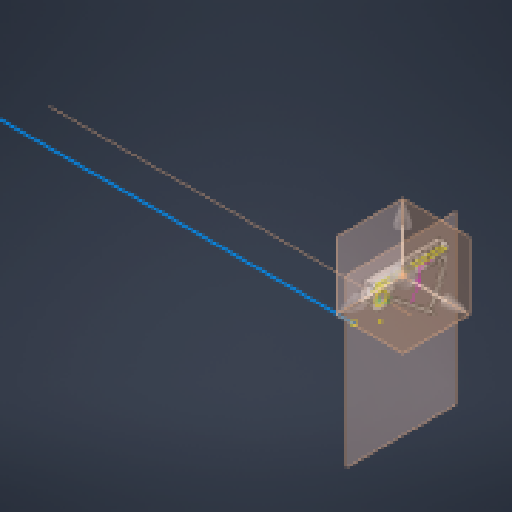
# Autodesk Inventor part: sensor arm v3
Saved by Autodesk Inventor 2025 (Build 290162000, 162)
## iProperties
Created: 2022-06-07
Part Number: sensor arm v3
Material: Generic
Document SubType Name: Modeling
Designer: micha
Density: 1 g/cm^3
Appearance: Default
Mass: 4.64954 g
Surface Area: 36.1007 cm^2
Volume: 4.64954 cm^3
Author: micha
Autodesk Inventor part; units mm, degrees
ref_plane "YZ Plane" through (0, 0, 0) normal (1, 0, 0) x (0, 1, 0)
ref_plane "XZ Plane" through (0, 0, 0) normal (0, 1, 0) x (-1, 0, 0)
ref_plane "XY Plane" through (0, 0, 0) normal (0, 0, 1) x (1, 0, 0)
ref_plane "Work Plane1" through (2.8939, -10.5569, -51.7376) normal (1, 0, 0) x (0, 0, -1)
sketch "Sketch1" plane through (2.8939, -10.5569, -51.7376) normal (1, 0, 0) x (0, 0, -1)
  line L0 (1, 38.5569) -> (1, -0.3026)
  spline S0 degree 2 poles (-6.3132, 4.7596) (-27.3933, 12.7232) (-66.3273, 26.8684) knots 1.083719 1.083719 1.083719 7.262987 7.262987 7.262987 weights 1.016219 1.054601 1.003399
  spline S1 degree 2 poles (-66, 24.0035) (-21.1228, 7.8362) (0, 0) knots 0 0 0 7.022956 7.022956 7.022956 weights 1 1.068995 1
  circle A0 centre (-63, 31.2793) radius 2.05
  circle A1 centre (-39, 31.2793) radius 2.05
  circle A2 centre (-27, 19.2793) radius 2.05
  circle A3 centre (-21, 25.2793) radius 2.05
  circle A4 centre (-15, 25.2793) radius 2.05
  circle A5 centre (-15, 19.2793) radius 2.05
  circle A6 centre (-21, 31.2793) radius 2.05
  circle A7 centre (-33, 19.2793) radius 2.05
  circle A8 centre (-45, 25.2793) radius 2.05
  circle A9 centre (-51, 31.2793) radius 2.05
  circle A10 centre (-51, 25.2793) radius 2.05
  circle A11 centre (-33, 25.2793) radius 2.05
  circle A12 centre (-27, 25.2793) radius 2.05
  circle A13 centre (-21, 19.2793) radius 2.05
  circle A14 centre (-15, 31.2793) radius 2.05
  circle A15 centre (-39, 25.2793) radius 2.05
  circle A16 centre (-15, 13.2793) radius 2.05
  circle A17 centre (-27, 31.2793) radius 2.05
  circle A18 centre (-33, 31.2793) radius 2.05
  circle A19 centre (-45, 31.2793) radius 2.05
  circle A20 centre (-57, 31.2793) radius 2.05
  line L1 (-6.3132, 20.0885) -> (-9, 20.0885)
  line L2 (-9, 20.0885) -> (-9, 22.0793)
  line L3 (-9, 22.0793) -> (-6.3132, 22.0793)
  line L4 (-6.3132, 22.0793) -> (-6.3132, 26.0885)
  line L5 (-6.3132, 26.0885) -> (-9, 26.0885)
  line L6 (-9, 26.0885) -> (-9, 28.0793)
  line L7 (-9, 28.0793) -> (-6.3132, 28.0793)
  line L8 (-6.3132, 28.0793) -> (-6.3132, 32.0885)
  line L9 (-6.3132, 32.0885) -> (-9, 32.0885)
  line L10 (-9, 32.0885) -> (-9, 34.0793)
  line L11 (-9, 34.0793) -> (-6.3132, 34.0793)
  line L12 (-6.3132, 34.0793) -> (-6.3132, 38.0885)
  line L13 (-6.3132, 38.0885) -> (-9, 38.0885)
  line L14 (-9, 38.0885) -> (-9, 38.5569)
  line L15 (-9, 38.5569) -> (-69, 38.5569)
  line L16 (-69, 38.5569) -> (-69, 26.0323)
  spline S2 degree 3 poles (-68.9282, 25.4918) (-68.9763, 25.6696) (-69, 25.8616) (-69, 26.0323) knots 0 0 0 0 1 1 1 1
  line L17 (-6.3132, 4.7596) -> (-6.3132, 8.0885)
  line L18 (-6.3132, 8.0885) -> (-9, 8.0885)
  line L19 (-9, 8.0885) -> (-9, 10.0793)
  line L20 (-9, 10.0793) -> (-6.3132, 10.0793)
  line L21 (-6.3132, 10.0793) -> (-6.3132, 14.0885)
  line L22 (-6.3132, 14.0885) -> (-9, 14.0885)
  line L23 (-9, 14.0885) -> (-9, 16.0793)
  line L24 (-9, 16.0793) -> (-6.3132, 16.0793)
  line L25 (-6.3132, 16.0793) -> (-6.3132, 20.0885)
  circle A21 centre (-51, 25.2793) radius 51
  line L26 (-69, 43.5569) -> (1, 43.5569)
  line L27 (0, 25.2793) -> (0, 43.5569)
  circle A22 centre (-63, 31.2793) radius 2.05
  circle A23 centre (-39, 31.2793) radius 2.05
  circle A24 centre (-27, 19.2793) radius 2.05
  circle A25 centre (-21, 25.2793) radius 2.05
  circle A26 centre (-15, 25.2793) radius 2.05
  circle A27 centre (-15, 19.2793) radius 2.05
  circle A28 centre (-21, 31.2793) radius 2.05
  circle A29 centre (-33, 19.2793) radius 2.05
  circle A30 centre (-45, 25.2793) radius 2.05
  circle A31 centre (-51, 31.2793) radius 2.05
  circle A32 centre (-51, 25.2793) radius 2.05
  circle A33 centre (-33, 25.2793) radius 2.05
  circle A34 centre (-27, 25.2793) radius 2.05
  circle A35 centre (-21, 19.2793) radius 2.05
  circle A36 centre (-15, 31.2793) radius 2.05
  circle A37 centre (-39, 25.2793) radius 2.05
  circle A38 centre (-15, 13.2793) radius 2.05
  circle A39 centre (-27, 31.2793) radius 2.05
  circle A40 centre (-33, 31.2793) radius 2.05
  circle A41 centre (-45, 31.2793) radius 2.05
  circle A42 centre (-57, 31.2793) radius 2.05
  line L28 (0, 3.2928) -> (0, 0)
  line L29 (-66, 43.5569) -> (-66, 24.0035)
  line L30 (-7.9338, 43.5569) -> (-66, 43.5569)
  line L31 (1, 3.5569) -> (1, 2.9251)
  spline S3 degree 2 poles (0, 3.2928) (0.5038, 3.1076) (1, 2.9251) knots 0 0 0 1 1 1 weights 1.002419 1.001235 1
  line L32 (-5.5888, 2.0667) -> (-8.7079, -13.6264)
  line L33 (-51, 25.2793) -> (1.0658, -16.3025)
  line L34 (-49.7207, 26.8812) -> (1, -13.6264)
  circle A43 centre (-51, 25.2793) radius 57.952
  circle A44 centre (-51, 25.2793) radius 49.5
  circle A45 centre (-51, 25.2793) radius 5
  line L35 (-51, 30.2793) -> (1, 30.2793)
  line L36 (-51, 28.5561) -> (1, 28.5561)
  line L37 (-6, 27.6203) -> (1, 27.6203)
  line L38 (1, 30.1203) -> (1, 27.6203)
  line L39 (1, 30.1203) -> (-7, 30.1203)
  line L40 (-7, 24.1203) -> (-7, 30.1203)
  line L41 (1, 24.1203) -> (-7, 24.1203)
  line L42 (1, 26.6203) -> (1, 24.1203)
  line L43 (1, 26.6203) -> (-6, 26.6203)
  line L44 (-6, 26.6203) -> (-6, 27.6203)
  line L45 (1, 43.5569) -> (1, -27.3438)
  circle A46 centre (-51, 25.2793) radius 3
  line L46 (-7.9338, 3.5569) -> (1, 3.5569)
  spline S4 degree 3 poles (-68.9282, 25.4918) (-68.9051, 25.5773) (-68.8768, 25.6596) (-68.7507, 25.9672) (-68.5854, 26.218) (-68.2351, 26.5719) (-67.989, 26.7385) (-67.5342, 26.9287) (-67.2454, 26.9869) (-67, 26.9869) (-66.8321, 26.9869) (-66.6438, 26.9597) (-66.4687, 26.9138) knots 0 0 0 0 0.082605 0.082605 0.334613 0.334613 0.583858 0.583858 0.830936 0.830936 0.830936 1 1 1 1
  line L47 (-67.3682, 24.0029) -> (-66.4687, 26.9138)
  spline S5 degree 2 poles (-67.3682, 24.0029) (-63.8358, 22.7167) (-60.4985, 21.4988) knots 0.11627 0.11627 0.11627 0.626298 0.626298 0.626298 weights 1.002483 1.007844 1.012449
  line L48 (-60.1926, 22.4888) -> (-60.4985, 21.4988)
  line L49 (-60.273, 22.4962) -> (-60.1926, 22.4888)
  line L50 (-61.0288, 24.942) -> (-60.273, 22.4962)
  spline S6 degree 2 poles (-57.0533, 23.4947) (-59.0095, 24.2073) (-61.0288, 24.942) knots 0 0 0 1 1 1 weights 1.014246 1.01214 1.009793
  line L51 (-57.4032, 22.3623) -> (-57.0533, 23.4947)
  line L52 (-56.7087, 20.1148) -> (-57.4032, 22.3623)
  spline S7 degree 2 poles (-56.7087, 20.1148) (-54.1005, 19.1616) (-51.6095, 18.2493) knots 0 0 0 1 1 1 weights 1.017547 1.020956 1.023858
  line L53 (-50.7041, 21.1795) -> (-51.6095, 18.2493)
  spline S8 degree 2 poles (-47.3081, 19.939) (-48.981, 20.5505) (-50.7041, 21.1795) knots 0 0 0 1 1 1 weights 1.023609 1.022223 1.020626
  line L54 (-46.1695, 16.2542) -> (-47.3081, 19.939)
  spline S9 degree 2 poles (-46.1695, 16.2542) (-44.6707, 15.7038) (-43.2153, 15.1685) knots 0 0 0 1 1 1 weights 1.029758 1.031251 1.032536
  line L55 (-42.3067, 18.1089) -> (-43.2153, 15.1685)
  spline S10 degree 2 poles (-37.3514, 16.2915) (-39.7706, 17.1799) (-42.3067, 18.1089) knots 0 0 0 1 1 1 weights 1.030206 1.029053 1.02736
  line L56 (-36.2059, 12.5846) -> (-37.3514, 16.2915)
  spline S11 degree 2 poles (-36.2059, 12.5846) (-35.7451, 12.4143) (-35.2889, 12.2456) knots 0 0 0 1 1 1 weights 1.037681 1.037944 1.038183
  line L57 (-34.3765, 15.1982) -> (-35.2889, 12.2456)
  spline S12 degree 2 poles (-31.8369, 14.2634) (-33.0902, 14.7251) (-34.3765, 15.1982) knots 0 0 0 1 1 1 weights 1.032167 1.031883 1.031435
  line L58 (-32.7507, 11.3063) -> (-31.8369, 14.2634)
  spline S13 degree 2 poles (-32.7507, 11.3063) (-31.3433, 10.7849) (-29.9802, 10.2787) knots 0 0 0 1 1 1 weights 1.039335 1.039874 1.040168
  line L59 (-31.1312, 14.0034) -> (-29.9802, 10.2787)
  spline S14 degree 2 poles (-27.9388, 12.8256) (-29.5079, 13.4052) (-31.1312, 14.0034) knots 0 0 0 1 1 1 weights 1.03266 1.032626 1.032315
  line L60 (-27.3534, 10.9314) -> (-27.9388, 12.8256)
  line L61 (-26.888, 12.4374) -> (-27.3534, 10.9314)
  spline S15 degree 2 poles (-24.3498, 11.4984) (-25.601, 11.9617) (-26.888, 12.4374) knots 0 0 0 1 1 1 weights 1.03236 1.032601 1.032651
  line L62 (-25.2685, 8.5253) -> (-24.3498, 11.4984)
  spline S16 degree 2 poles (-25.2685, 8.5253) (-23.1143, 7.7218) (-21.0732, 6.9569) knots 0 0 0 1 1 1 weights 1.040431 1.040189 1.039256
  line L63 (-22.2343, 10.7144) -> (-21.0732, 6.9569)
  spline S17 degree 2 poles (-17.2807, 8.8727) (-19.6843, 9.7684) (-22.2343, 10.7144) knots 2.532276 2.532276 2.532276 3.127294 3.127294 3.127294 weights 1.029291 1.030965 1.031808
  line L64 (-18.0732, 6.3082) -> (-17.2807, 8.8727)
  line L65 (-17.9038, 5.7667) -> (-18.0732, 6.3082)
  spline S18 degree 2 poles (-17.9038, 5.7667) (-15.9349, 5.0258) (-14.071, 4.3204) knots 0 0 0 1 1 1 weights 1.037347 1.035864 1.033687
  line L66 (-13.4423, 6.3549) -> (-14.071, 4.3204)
  line L67 (-13.8213, 7.5812) -> (-13.4423, 6.3549)
  spline S19 degree 2 poles (-10.6072, 6.3767) (-12.1801, 6.9674) (-13.8213, 7.5812) knots 0 0 0 1 1 1 weights 1.022735 1.024771 1.02639
  line L68 (-10.6139, 6.3549) -> (-10.6072, 6.3767)
  line L69 (-9.4416, 2.5612) -> (-10.6139, 6.3549)
  spline S20 degree 2 poles (-9.4416, 2.5612) (-8.5985, 2.2395) (-7.7778, 1.9252) knots 0 0 0 1 1 1 weights 1.026979 1.025506 1.023872
  line L70 (-6.8404, 4.9587) -> (-7.7778, 1.9252)
  spline S21 degree 2 poles (-6.3132, 4.7596) (-6.5758, 4.8589) (-6.8404, 4.9587) knots 0 0 0 1 1 1 weights 1.016219 1.01668 1.017128
  spline S22 degree 2 poles (-47.8503, 17.4555) (-47.0907, 17.181) (-46.3417, 16.9102) knots 0 0 0 1 1 1 weights 1.022634 1.023401 1.024117
  spline S23 degree 2 poles (-0.7385, 0.2738) (-0.3669, 0.1361) (0, 0) knots 0 0 0 1 1 1 weights 1.002208 1.001122 1
  spline S24 degree 2 poles (-0.7385, 0.2738) (-1.5648, 0.5801) (-2.4148, 0.8945) knots 0 0 0 1 1 1 weights 1.005252 1.007625 1.009817
  spline S25 degree 2 poles (-4.9534, 1.8323) (-3.6579, 1.3544) (-2.4148, 0.8945) knots 0 0 0 1 1 1 weights 1.01307 1.010167 1.006872
  spline S26 degree 2 poles (-4.9534, 1.8323) (-5.0001, 1.8495) (-5.0468, 1.8668) knots 0 0 0 1 1 1 weights 1.015865 1.015967 1.016069
  spline S27 degree 2 poles (-8.2385, 3.0424) (-6.6033, 2.4409) (-5.0468, 1.8668) knots 0 0 0 1 1 1 weights 1.019681 1.016766 1.013279
  spline S28 degree 2 poles (-8.2385, 3.0424) (-8.4827, 3.1322) (-8.7287, 3.2226) knots 0 0 0 1 1 1 weights 1.022285 1.022707 1.023117
  spline S29 degree 2 poles (-11.2688, 4.1555) (-9.9751, 3.6808) (-8.7287, 3.2226) knots 0 0 0 1 1 1 weights 1.024514 1.022693 1.020541
  spline S30 degree 2 poles (-11.2688, 4.1555) (-12.1147, 4.4658) (-12.9815, 4.7835) knots 0 0 0 1 1 1 weights 1.026945 1.02809 1.029093
  spline S31 degree 2 poles (-17.9571, 6.6037) (-15.3856, 5.6644) (-12.9815, 4.7835) knots 4.545675 4.545675 4.545675 5.174639 5.174639 5.174639 weights 1.031505 1.029685 1.026759
  spline S32 degree 2 poles (-17.9571, 6.6037) (-19.6666, 7.2282) (-21.4541, 7.8799) knots 0 0 0 1 1 1 weights 1.033564 1.034685 1.035312
  spline S33 degree 2 poles (-25.0396, 9.186) (-23.2077, 8.5192) (-21.4541, 7.8799) knots 0 0 0 1 1 1 weights 1.034382 1.034148 1.03344
  spline S34 degree 2 poles (-25.0396, 9.186) (-27.4467, 10.0621) (-29.9959, 10.9881) knots 3.443887 3.443887 3.443887 3.981642 3.981642 3.981642 weights 1.036069 1.036254 1.035617
  spline S35 degree 2 poles (-31.3054, 11.4637) (-30.6459, 11.2242) (-29.9959, 10.9881) knots 0 0 0 1 1 1 weights 1.033862 1.034046 1.034176
  spline S36 degree 2 poles (-31.3054, 11.4637) (-31.5323, 11.546) (-31.7603, 11.6288) knots 0 0 0 1 1 1 weights 1.035239 1.035165 1.035085
  spline S37 degree 2 poles (-33.4388, 12.2379) (-32.5919, 11.9307) (-31.7603, 11.6288) knots 0 0 0 1 1 1 weights 1.033138 1.033475 1.033729
  spline S38 degree 2 poles (-33.4388, 12.2379) (-35.6339, 13.0343) (-37.9355, 13.8682) knots 0 0 0 1 1 1 weights 1.034414 1.033438 1.0319
  spline S39 degree 2 poles (-39.3424, 14.3777) (-38.6339, 14.1212) (-37.9355, 13.8682) knots 0 0 0 1 1 1 weights 1.029908 1.030394 1.030829
  spline S40 degree 2 poles (-39.3424, 14.3777) (-40.1336, 14.6643) (-40.9376, 14.9553) knots 0 0 0 1 1 1 weights 1.030917 1.03034 1.029698
  spline S41 degree 2 poles (-42.8319, 15.6409) (-41.8759, 15.295) (-40.9376, 14.9553) knots 0 0 0 1 1 1 weights 1.027259 1.028053 1.02876
  spline S42 degree 2 poles (-42.8319, 15.6409) (-44.5572, 16.2651) (-46.3417, 16.9102) knots 0 0 0 1 1 1 weights 1.028117 1.026614 1.02483
  spline S43 degree 2 poles (-47.8503, 17.4555) (-49.2326, 17.9551) (-50.651, 18.4673) knots 0 0 0 1 1 1 weights 1.023286 1.021839 1.02023
  spline S44 degree 2 poles (-52.7716, 19.2331) (-51.7012, 18.8466) (-50.651, 18.4673) knots 0 0 0 1 1 1 weights 1.017303 1.01854 1.019688
  spline S45 degree 2 poles (-52.7716, 19.2331) (-53.9932, 19.6741) (-55.2416, 20.1246) knots 0 0 0 1 1 1 weights 1.017764 1.01631 1.01474
  spline S46 degree 2 poles (-56.8566, 20.7073) (-56.0435, 20.414) (-55.2416, 20.1246) knots 0 0 0 1 1 1 weights 1.012371 1.013395 1.014371
  spline S47 degree 2 poles (-56.8566, 20.7073) (-58.8593, 21.4298) (-60.9319, 22.177) knots 0 0 0 1 1 1 weights 1.012682 1.010099 1.00723
  spline S48 degree 2 poles (-63.2903, 23.0271) (-62.0997, 22.598) (-60.9319, 22.177) knots 0 0 0 1 1 1 weights 1.003834 1.005493 1.007062
  spline S49 degree 2 poles (-63.2903, 23.0271) (-63.9732, 23.2732) (-64.6637, 23.522) knots 0 0 0 1 1 1 weights 1.003923 1.002951 1.00195
  spline S50 degree 2 poles (-66, 24.0035) (-65.3283, 23.7615) (-64.6637, 23.522) knots 0 0 0 1 1 1 weights 1 1.000967 1.001907
  line L71 (-7.9338, 43.5569) -> (-7.9338, 3.5569)
  point P0 (-51.7376, 10.5569)
  point P1 (-4.4661, -9.261)
  point P2 (-5.717, -10.8854)
  point P3 (-11.0752, -3.9826)
  point P4 (-46.1572, 24.0352)
  point P5 (-47.2234, 28.5561)
  point P6 (-1.6086, 28.5561)
  point P7 (-0.2303, 30.1203)
  point P8 (-6.3132, 30.1203)
  point P9 (-6.3132, 30.2793)
  point P10 (-49.2104, 30.2793)
  point P11 (-49.3883, 30.0124)
  point P12 (-47.0931, 22.1591)
  point P13 (-11.1492, -6.5471)
  point P14 (-0.2457, 30.2793)
extrude "Thickness" add sketch "Sketch1" along normal mid plane 3 contours A21 L39 A44 L35 | A21 L36 A44 L39 | A44 L39 L8 L35 | L33 A44 L34 A21 | A21 L37 A44 L36 | A44 L36 L8 L39 | L8 L39 L40 L36 L71 L35 | L34 A44 S1 A21 | L33 L57 S1 L58 S13 L59 L34 A44 | A21 L43 A44 L37 | L8 L36 L40 L39 | L71 L36 A45 A9 L35 A19 A1 A18 A17 A6 A14 | S1 A44 L46 A21 | L33 S1 L57 | L41 A44 L43 A21 | A21 L46 A44 L41 | A14 L35 | S1 L59 L34 | L33 L56 S0 L34 L57 S1 | L57 L34 L58 S1 | A45 A8 L34 A46 L33 S0 A9 | L59 S1 L58 L34 | L33 S0 L56 | A6 L35 | A45 L34 A8 | A9 A45 | L59 S13 L58 S1 | L33 A45 A8 L34 S0 | L34 A45 A8 | A8 A45 L33 A46 L34 | A8 A45 L34 | A17 L35 | A46 L33 A10 L34 | L34 A10 L33 A46 | S0 L53 A45 | L35 A19 | A45 L53 S0 | A18 L35 | L35 A1 picked at (-15.4743, 29.9145) picked at (-21.4743, 29.9145) picked at (-46.3486, 25.5853) picked at (-46.6382, 24.3353) picked at (-45.6216, 23.5252) picked at (-27.4743, 29.9145) picked at (-44.8638, 29.6994) picked at (-32.9196, 29.6737) picked at (-38.8638, 29.6994)
sketch "Sketch2" plane through (1.3939, 19.7224, -2.5271) normal (0, 1, 0) x (1, 0, 0)
  line L0 (0, 0) -> (0, 48.9648) projected
  line L1 (0, 0) -> (3, 0) projected
  line L2 (3, 48.9648) -> (3, 0) projected
  line L3 (0, 48.9648) -> (3, 48.9648) projected
  line L4 (0, 2.1174) -> (0, -0.1779) projected
  line L5 (0, 2.1174) -> (3, 2.1174) projected
  line L6 (3, -0.1779) -> (3, 2.1174) projected
  line L7 (0, -0.1779) -> (3, -0.1779) projected
  line L8 (3, -6.7896) -> (3, 2.1174) projected
  line L9 (0, 49.2104) -> (0, 38.0612) projected
  line L10 (3, -6.7896) -> (0, -6.7896)
  line L11 (0, -6.7896) -> (0, 49.2104)
  line L12 (0, 49.2104) -> (3, 49.2104)
  line L13 (3, 49.2104) -> (3, -6.7896)
  point P0 (-1.3939, -2.5271)
  constraints: 8 end point, 2 parallel, 1 horizontal, 1 perpendicular
sketch "Sketch3" plane through (4.3939, -10.5569, -51.7376) normal (1, 0, 0) x (0, 0, -1)
  arc A0 (-11.1492, -6.5471) -> (-0.2457, 30.2793) centre (-51, 25.2793) ccw projected
  line L0 (-0.2457, 30.2793) -> (-47.7223, 30.2793)
  line L1 (-47.7223, 30.2793) -> (-47.7223, 24.2793)
  line L2 (-47.7223, 24.2793) -> (-0.2457, 24.2793)
  line L3 (-0.2457, 24.2793) -> (-0.2457, 30.2793)
  point P0 (-51.7376, 10.5569)
  dimension "d10" = 6
  constraints: 8 end point, 2 parallel, 1 horizontal, 1 perpendicular
  measures "d10" distance between parallel lines of L2 L0
extrude "sensor weight" [suppressed]
sketch "Sketch4" plane through (1.3939, 19.7224, -2.5271) normal (0, 1, 0) x (1, 0, 0)
  line L0 (0, 0) -> (3, 0) projected
  line L1 (3, 48.9648) -> (3, 0) projected
  line L2 (0, 48.9648) -> (3, 48.9648) projected
  line L3 (0, 0) -> (0, 48.9648) projected
  line L4 (3, 45.6506) -> (0, 45.6506)
  line L5 (0, 47.6019) -> (0, 1.987) projected
  line L6 (11.5, 52.7104) -> (-8.5, 52.7104) projected
  line L7 (-8.5, 52.7104) -> (-8.5, 50.2104) projected
  line L8 (-5.5, 50.2104) -> (-8.5, 50.2104) projected
  line L9 (-1.5, 50.2104) -> (-5.5, 50.2104) projected
  line L10 (4.5, 50.2104) -> (-1.5, 50.2104) projected
  line L11 (8.3, 41.7104) -> (4.5, 41.7104) projected
  line L12 (8.3, 50.2104) -> (8.3, 41.7104) projected
  line L13 (11.5, 50.2104) -> (8.3, 50.2104) projected
  line L14 (11.5, 52.7104) -> (11.5, 50.2104) projected
  line L15 (-1.5, 50.2104) -> (-5.5, 50.2104) projected
  line L16 (-1.5, 41.7104) -> (-5.5, 41.7104) projected
  line L17 (3, 48.9648) -> (3, 0) projected
  line L18 (0, 0) -> (0, 48.9648) projected
  line L19 (-2.5, -6.7896) -> (5.5, -6.7896)
  line L20 (5.5, -6.7896) -> (5.5, 48.9648)
  line L21 (5.5, 48.9648) -> (-2.5, 48.9648)
  line L22 (-2.5, 48.9648) -> (-2.5, -6.7896)
  line L23 (-2.5, -6.7896) -> (5.5, 48.9648) construction
  line L24 (5.5, -6.7896) -> (-2.5, 48.9648) construction
  line L25 (1.5, 64.6104) -> (1.5, -18.6896) projected
  line L26 (3, -6.7896) -> (0, -6.7896) projected
  line L27 (4.5, 50.2104) -> (4.5, 41.7104) projected
  line L28 (-1.5, 41.7104) -> (-1.5, 50.2104) projected
  line L29 (-5.5, 50.2104) -> (-5.5, 41.7104) projected
  point P0 (-1.3939, -2.5271)
  point P1 (1.5, 21.0876)
  point P2 (1.5, 48.9648)
  point P3 (1.5, 21.0876)
  point P4 (1.5, -6.7896)
  dimension "d29" = 8
  constraints: 14 end point, 7 midpoint, 3 point on line, 2 parallel, 2 perpendicular, 1 horizontal
  measures "d29" distance of L20.end L21.end
extrude "magnet mount and/or counterweight" add sketch "Sketch4" along normal blind 5 contours L3 L4 L25 L0 | L0 L25 L19 L22 L16 L28 L21 L3 | L25 L4 L1 L0 | L0 L1 L21 L27 L11 L20 L19 L25 | L25 L2 L1 L4 | L4 L3 L2 L25 | L21 L20 L11 L27 | L28 L16 L22 L21
sketch "Sketch5" plane through (1.3939, 24.7224, -2.5271) normal (0, 1, 0) x (1, 0, 0)
  line L0 (-2.5, -6.7896) -> (5.5, -6.7896) projected
  line L1 (3, 3.9648) -> (0, 3.9648) projected
  line L2 (1.5, 3.9648) -> (1.5, 48.9648)
  line L3 (-2.5, 48.9648) -> (-2.5, -6.7896) projected
  line L4 (-2.5, 21.0876) -> (5.5, 21.0876)
  line L5 (5.5, -6.7896) -> (5.5, 48.9648) projected
  circle A0 centre (1.5, 44.6266) radius 1.45
  circle A1 centre (1.5, 39.6266) radius 1.45
  circle A2 centre (1.5, 34.6266) radius 1.45
  circle A3 centre (1.5, 29.6266) radius 1.45
  circle A4 centre (1.5, 24.6266) radius 1.45
  circle A5 centre (1.5, 19.6266) radius 1.45
  point P0 (-1.3939, -2.5271)
  dimension "d19" = 2.9
  dimension "d22" = 5
  constraints: 6 centre point, 4 end point, 3 midpoint, 1 parallel, 1 point on line, 1 vertical, 11 other
  measures "d19" diameter of A0
  measures "d22" distance of A0.centre A1.centre
extrude "Extrusion4" cut sketch "Sketch5" against normal up to surface (6.7232 mm away) contours A5 L2 | L2 A5 | A4 L2 | L2 A4 | A3 L2 | L2 A3 | A2 L2 | L2 A2 | A1 L2 | L2 A1 | A0 L2 | L2 A0
sketch "Sketch6" plane through (1.3939, 24.7224, -2.5271) normal (0, 1, 0) x (1, 0, 0)
  line L0 (-2.5, -6.7896) -> (5.5, -6.7896) projected
  line L1 (-2.5, 48.9648) -> (-2.5, -6.7896) projected
  line L2 (5.5, -6.7896) -> (-2.5, -6.7896)
  line L3 (-2.5, -6.7896) -> (-2.5, 8.2104)
  line L4 (-2.5, 8.2104) -> (5.5, 8.2104)
  line L5 (5.5, 8.2104) -> (5.5, -6.7896)
  point P0 (-1.3939, -2.5271)
  dimension "d30" = 15
  constraints: 8 end point, 2 parallel, 1 horizontal, 1 perpendicular, 1 point on line
  measures "d30" distance of L2.end L3.end
extrude "Extrusion5" add sketch "Sketch6" against normal blind 10
sketch "Sketch7" plane through (-1.1061, 24.7224, 4.2624) normal (0, 0, 1) x (1, 0, 0)
  line L0 (8, 0) -> (8, -10) projected
  line L1 (0, 0) -> (8, 0) projected
  line L2 (0, -10) -> (0, 0) projected
  line L3 (2.5, -10) -> (0, -10) projected
  line L4 (2.5, -10) -> (5.5, -10) projected
  line L5 (8, -10) -> (5.5, -10) projected
  line L6 (5.5, -15) -> (5.5, -10) projected
  line L7 (2.5, -10) -> (2.5, -15) projected
  line L8 (0, 0) -> (8, 0) projected
  line L9 (2.5, -10) -> (5.5, -10)
  line L10 (5.5, -10) -> (5.5, 0)
  line L11 (5.5, 0) -> (2.5, 0)
  line L12 (2.5, 0) -> (2.5, -10)
  line L13 (0, 0) -> (2.5, 0)
  line L14 (2.5, 0) -> (2.5, -10)
  line L15 (2.5, -10) -> (0, -10)
  line L16 (0, -10) -> (0, 0)
  line L17 (8, -10) -> (5.5, -10) projected
  line L18 (5.5, -10) -> (8, -10)
  line L19 (8, -10) -> (8, 0)
  line L20 (8, 0) -> (5.5, 0)
  line L21 (5.5, 0) -> (5.5, -10)
  point P0 (1.1061, -24.7224)
  point P1 (5.5, -13.1202)
  point P2 (2.5, -13.1202)
  point P3 (2.5, 0)
  point P4 (5.5, 0)
  constraints: 24 end point, 6 parallel, 3 horizontal, 3 perpendicular, 1 point on line
extrude "thin near bearing" [suppressed]
sketch "Sketch8" plane through (1.3939, 14.7224, -2.5271) normal (0, -1, 0) x (1, 0, 0)
  line L0 (-2.5, 6.7896) -> (-2.5, -8.2104) projected
  line L1 (-2.5, -8.2104) -> (5.5, -8.2104) projected
  line L2 (5.5, -8.2104) -> (5.5, 6.7896) projected
  line L3 (0, -3.2104) -> (3, -3.2104) projected
  line L4 (0, -8.2104) -> (-2.5, -8.2104) projected
  line L5 (5.5, 6.7896) -> (5.5, -48.9648) projected
  line L6 (-2.5, -8.2104) -> (5.5, -8.2104)
  line L7 (5.5, -8.2104) -> (5.5, -3.2104)
  line L8 (5.5, -3.2104) -> (-2.5, -3.2104)
  line L9 (-2.5, -3.2104) -> (-2.5, -8.2104)
  line L10 (-2.5, -8.2104) -> (5.5, -8.2104)
  line L11 (5.5, -8.2104) -> (5.5, -2.7104)
  line L12 (5.5, -2.7104) -> (-2.5, -2.7104)
  line L13 (-2.5, -2.7104) -> (-2.5, -8.2104)
  line L14 (0, -0.2604) -> (0, -3.2104) projected
  line L15 (3, -0.2604) -> (0, -0.2604) projected
  line L16 (3, -3.2104) -> (3, -0.2604) projected
  line L17 (3, 3.8396) -> (3, 6.7896) projected
  line L18 (0, 3.8396) -> (3, 3.8396) projected
  line L19 (0, 6.7896) -> (0, 3.8396) projected
  line L20 (0, 6.7896) -> (-2.5, 6.7896) projected
  line L21 (5.5, 6.7896) -> (3, 6.7896) projected
  point P0 (-1.3939, 2.5271)
  point P1 (0, -2.7104)
  point P2 (3, -2.7104)
  dimension "d37" = 5.5
  constraints: 16 end point, 4 parallel, 2 horizontal, 2 perpendicular
  measures "d37" distance of L11.end L10.end
extrude "Extrusion7" [suppressed]
sketch "Sketch9" plane through (1.3939, -10.5569, -51.7376) normal (-1, 0, 0) x (0, 0, 1)
  arc A0 (51, 30.2793) -> (49.3883, 30.0124) centre (51, 25.2793) ccw projected
  circle A1 centre (51, 25.2793) radius 4.65
  point P0 (51.7376, 10.5569)
  point P1 (47.0931, 22.1591)
  point P2 (56, 25.2793)
  dimension "d38" = 9.3
  constraints: 1 centre point, 1 coincident
  measures "d38" diameter of A1
sketch "Sketch10" plane through (2.8939, -10.5569, -51.7376) normal (1, 0, 0) x (0, 0, -1)
  line L0 (-48.95, 25.2793) -> (-53.05, 25.2793) projected
  circle A0 centre (-51, 25.2793) radius 8
  circle A1 centre (-51, 25.2793) radius 3
  point P0 (-51.7376, 10.5569)
  dimension "d39" = 16
  dimension "d40" = 6
  constraints: 2 centre point, 1 coincident, 1 midpoint
  measures "d39" diameter of A0
  measures "d40" diameter of A1
extrude "Extrusion8" add sketch "Sketch10" along normal mid plane 8
sketch "Sketch11" plane through (6.8939, 19.7224, -51.4919) normal (1, 0, 0) x (0, 0, -1)
  circle A0 centre (-50.7543, -5) radius 4.5 projected
  circle A1 centre (-50.7543, -5) radius 4.6
  point P0 (-51.4919, -19.7224)
  dimension "d46" = 9.2
  constraints: 1 centre point, 1 coincident
  measures "d46" diameter of A1
extrude "Extrusion9" cut sketch "Sketch9" along normal through all both and the other way through all
sketch "Sketch12" plane through (2.8939, -10.5569, -51.7376) normal (1, 0, 0) x (0, 0, -1)
  line L0 (-7, 24.1203) -> (-1.182, 24.1203)
  line L1 (-1.182, 24.1203) -> (-1.182, 29.9482)
  line L2 (-1.182, 29.9482) -> (-7, 29.9482)
  line L3 (-7, 29.9482) -> (-7, 24.1203)
  line L4 (-8, 22.1203) -> (-1.182, 22.1203)
  line L5 (-1.182, 22.1203) -> (-1.182, 30.7039)
  line L6 (-1.182, 30.7039) -> (-8, 30.7039)
  line L7 (-8, 30.7039) -> (-8, 22.1203)
  point P0 (-51.7376, 10.5569)
  point P1 (-1.6086, 28.5561)
  dimension "d64" = 2
  dimension "d65" = 1
  constraints: 16 end point, 4 horizontal, 4 parallel, 2 perpendicular, 2 vertical, 1 point on line, 1 other
  measures "d64" distance between parallel lines of L4 L0
  measures "d65" distance between parallel lines of L7 L3
extrude "sensor flag" add sketch "Sketch12" along normal mid plane 3 contours L3 L2 L1 L0
sketch "Sketch13" plane through (1.3939, -10.5569, -51.7376) normal (-1, 0, 0) x (0, 0, 1)
  line L0 (1.5136, 24.1203) -> (7, 24.1203) projected
  line L1 (7, 24.1203) -> (7, 28.5561) projected
  line L2 (7, 28.5561) -> (41, 28.5561) projected
  line L3 (41, 28.5561) -> (41, 30.2793) projected
  line L4 (41, 30.2793) -> (0.2457, 30.2793) projected
  arc A0 (0.2457, 30.2793) -> (11.1492, -6.5471) centre (51, 25.2793) ccw projected
  line L5 (11.1492, -6.5471) -> (44.7489, 20.2869) projected
  arc A1 (43.6783, 22.0555) -> (44.7489, 20.2869) centre (51, 25.2793) ccw projected
  line L6 (43.6783, 22.0555) -> (11.0752, -3.9826) projected
  arc A2 (1.5136, 24.1203) -> (11.0752, -3.9826) centre (51, 25.2793) ccw projected
  line L7 (44.7489, 20.2869) -> (11.1492, -6.5471) projected
  line L8 (44.7489, 20.2869) -> (5.717, -10.8854)
  circle A3 centre (51, 25.2793) radius 4.65 projected
  circle A4 centre (51, 25.2793) radius 57.952
  line L9 (11.0752, -3.9826) -> (43.6783, 22.0555) projected
  line L10 (43.6783, 22.0555) -> (4.4661, -9.261)
  line L11 (0, 3.2928) -> (0, 0) projected
  line L12 (0, 0) -> (51, 25.2793)
  circle A5 centre (51, 25.2793) radius 55.952
  point P0 (51.7376, 10.5569)
  point P1 (-1, -0.3026)
  point P2 (9.9022, -4.9195)
  point P3 (11.1492, -6.5471)
  point P4 (6.0299, -8.0121)
  point P5 (7.2798, -9.6373)
  dimension "d54" = 56.9214
  dimension "d55" = 115.904
  dimension "d56" = 2
  constraints: 6 end point, 3 point on circle, 2 centre point, 2 coincident, 1 point on line, 1 other
  measures "d54" distance of L11.end L12.end
  measures "d55" diameter of A4
  measures "d56" radial gap between concentric circles of A4 A5
extrude "sensor arm extension" add sketch "Sketch13" against normal up to surface (3 mm away) contours A0 L8 A5 L10
sketch "Sketch14" plane through (1.3939, 19.7224, -2.5271) normal (0, -1, 0) x (1, 0, 0)
  line L0 (-1.5, -50.2104) -> (-1.5, -41.7104) projected
  line L1 (-5.5, -41.7104) -> (-1.5, -41.7104) projected
  line L2 (-5.5, -41.7104) -> (-5.5, -50.2104) projected
  line L3 (-5.5, -50.2104) -> (-8.5, -50.2104) projected
  line L4 (-8.5, -52.7104) -> (-8.5, -50.2104) projected
  line L5 (-8.5, -52.7104) -> (11.5, -52.7104) projected
  line L6 (11.5, -52.7104) -> (11.5, -50.2104) projected
  line L7 (8.3, -50.2104) -> (11.5, -50.2104) projected
  line L8 (8.3, -50.2104) -> (8.3, -41.7104) projected
  line L9 (4.5, -41.7104) -> (8.3, -41.7104) projected
  line L10 (4.5, -41.7104) -> (4.5, -50.2104) projected
  line L11 (-1.5, -50.2104) -> (4.5, -50.2104) projected
  line L12 (-2.5, -48.9648) -> (-2.5, -8.2104) projected
  line L13 (5.5, -6.2104) -> (5.5, 9.7896) projected
  line L14 (-2.5, -40.7104) -> (5.5, -40.7104)
  line L15 (5.5, -40.7104) -> (5.5, -6.2104)
  line L16 (5.5, -6.2104) -> (-2.5, -6.2104)
  line L17 (-2.5, -6.2104) -> (-2.5, -40.7104)
  point P0 (-1.3939, 2.5271)
  point P1 (5.5, 6.7896)
  point P2 (-2.5, -8.2104)
  dimension "d57" = 1
  constraints: 8 end point, 2 parallel, 1 horizontal, 1 perpendicular, 1 point on line
  measures "d57" distance between parallel lines of L9 L14
extrude "Extrusion12" add sketch "Sketch14" along normal blind 3 contours L12 L17 L16 L15 L14
sketch "Sketch15" plane through (1.3939, 17.9992, -44.7376) normal (0, 0, 1) x (1, 0, 0)
  line L0 (0, 0) -> (3, 0) projected
  line L1 (0, -4.4358) -> (0, 0) projected
  line L2 (0, -4.4358) -> (3, -4.4358) projected
  line L3 (3, 0) -> (3, -4.4358) projected
  point P0 (-1.3939, -17.9992)
extrude "Extrusion13" add sketch "Sketch15" along normal blind 5
fillet "Fillet1" radius 1 2 edges at (4.3939, 19.7224, -47.3647) (1.3939, 19.7224, -47.3647)
fillet "Fillet2" radius 1 11 edges at (3.6439, 9.73, -6.9887) (2.1439, 9.73, -6.9887) (1.3939, 10.5796, -7.5813) (4.3939, 10.5796, -7.5813) (2.1439, 11.4986, -8.0592) (3.6439, 11.4986, -8.0592) (2.1439, -15.4764, -41.8354) (3.6439, -15.4764, -41.8354) (2.8939, -14.5396, -40.6623) (2.8939, -20.1943, -44.4578) (2.8939, -18.569, -45.7077)
fillet "Fillet3" radius 1 10 edges at (2.8939, 13.5634, -39.7376) (2.8939, 16.7224, -39.7376) (5.6439, 16.7224, -43.2376) (4.6868, 19.4295, -43.2376) (4.3939, 17.7224, -43.2376) (6.1439, 19.7224, -43.2376) (1.3939, 16.7224, -41.4876) (1.101, 19.4295, -43.2376) (-0.3561, 19.7224, -43.2376) (1.3939, 17.7224, -43.2376)
fillet_without_effect "Fillet4"
body "Solid1"
